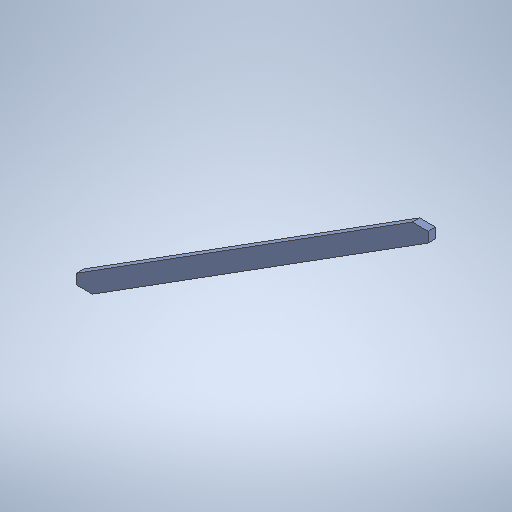
# Autodesk Inventor part: side2
Saved by Autodesk Inventor 2025.1 (Build 291241020, 241B)
## iProperties
Created: 2024-09-16
Part Number: side2
Material: Generic
Document SubType Name: Modeling
Designer: User
Density: 1 g/cm^3
Appearance: Default
Author: User
Autodesk Inventor part; units mm, degrees
ref_plane "YZ Plane" through (0, 0, 0) normal (1, 0, 0) x (0, 1, 0)
ref_plane "XZ Plane" through (0, 0, 0) normal (0, 1, 0) x (-1, 0, 0)
ref_plane "XY Plane" through (0, 0, 0) normal (0, 0, 1) x (1, 0, 0)
sketch "Sketch1" plane through (0, 0, 0) normal (0, 0, 1) x (1, 0, 0)
  line L0 (-914.4, 0) -> (914.4, 0) projected
  line L1 (-914.4, 2482.85) -> (-914.4, -2393.95) projected
  line L2 (914.4, -2393.95) -> (914.4, 2482.85) projected
  line L3 (-914.4, -1155.7) -> (914.4, -1155.7) projected
  line L4 (914.4, -52.5818) -> (-831.1936, -1155.7)
  line L5 (-914.4, -1103.1182) -> (831.1936, 0)
  line L6 (914.4, -52.5818) -> (914.4, 0)
  line L7 (914.4, 0) -> (831.1936, 0)
  line L8 (-914.4, -1103.1182) -> (-914.4, -1155.7)
  line L9 (-831.1936, -1155.7) -> (-914.4, -1155.7)
  point P0 (0, 0)
  constraints: 12 end point, 4 point on line, 3 collinear, 1 parallel, 1 perpendicular, 2 other
extrude "Extrusion1" add sketch "Sketch1" against normal blind 38.1 contours L0 L2 L4 L3 L1 L5
body "Solid1"
